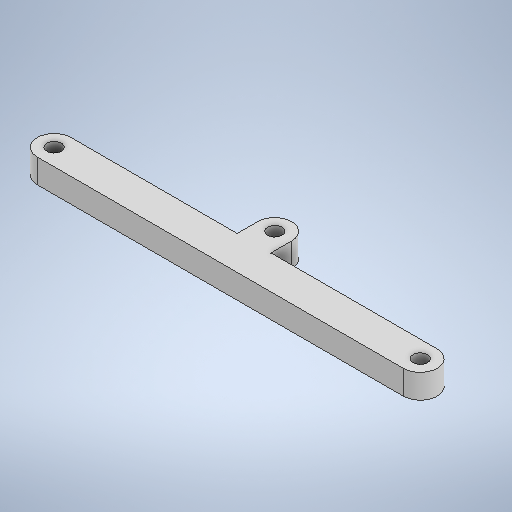
# Autodesk Inventor part: connector
Saved by Autodesk Inventor 2026 (Build 300175050, 175E)
## iProperties
Created: 2025-05-24
Part Number: connector
Material: Generic
Document SubType Name: Modeling
Designer: omiye
Density: 1 g/cm^3
Appearance: Default
Author: omiye
Autodesk Inventor part; units mm, degrees
ref_plane "YZ Plane" through (0, 0, 0) normal (1, 0, 0) x (0, 1, 0)
ref_plane "XZ Plane" through (0, 0, 0) normal (0, 1, 0) x (-1, 0, 0)
ref_plane "XY Plane" through (0, 0, 0) normal (0, 0, 1) x (1, 0, 0)
sketch "Sketch1" plane through (0, 0, 0) normal (0, 1, 0) x (-1, 0, 0)
  line L0 (-19, -3.5) -> (-19, 3.5)
  line L1 (-19, 3.5) -> (19, 3.5)
  line L2 (19, 3.5) -> (19, -3.5)
  line L3 (19, -3.5) -> (-19, -3.5)
  line L4 (-19, -3.5) -> (19, 3.5) construction
  line L5 (-19, 3.5) -> (19, -3.5) construction
  circle A0 centre (19, 0) radius 1.5
  line L6 (19, 3.5) -> (22.5, 3.5)
  line L7 (22.5, 3.5) -> (22.5, -3.5)
  line L8 (22.5, -3.5) -> (19, -3.5)
  line L9 (19, -3.5) -> (19, 3.5)
  line L10 (-19, 0) -> (-19, -7.8)
  line L11 (-22.5, 14.8) -> (-22.5, -7.8)
  line L12 (-22.5, -7.8) -> (-15.5, -7.8)
  line L13 (-15.5, -7.8) -> (-15.5, 14.8)
  line L14 (-15.5, 14.8) -> (-22.5, 14.8)
  line L15 (-22.5, 14.8) -> (-15.5, -7.8) construction
  line L16 (-22.5, -7.8) -> (-15.5, 14.8) construction
  line L17 (-19, 3.5) -> (-22.5, 3.5)
  circle A1 centre (-19, -7.8) radius 1.5
  line L18 (-15.5, -7.8) -> (-22.5, -7.8)
  line L19 (-22.5, -7.8) -> (-22.5, -11.3)
  line L20 (-22.5, -11.3) -> (-15.5, -11.3)
  line L21 (-15.5, -11.3) -> (-15.5, -7.8)
  point P0 (0, 0)
  point P1 (-22.5, -7.8)
  point P2 (-15.5, -3.5)
  dimension "d0" = 7
  dimension "d1" = 38
  dimension "d2" = 3
  dimension "d3" = 3.5
  dimension "d4" = 7.8
  dimension "d5" = 7
  dimension "d6" = 3
  dimension "d7" = 3.5
  constraints: 44 end point, 9 parallel, 7 midpoint, 4 perpendicular, 2 centre point, 2 horizontal, 1 coincident, 1 point on line, 1 vertical
  measures "d0" distance of L0.start L0.end
  measures "d1" distance of L0.end L1.end
  measures "d2" diameter of A0
  measures "d3" distance of L7.end L8.end
  measures "d4" distance of L10.start L10.end
  measures "d5" distance of L12.end L11.end
  measures "d6" diameter of A1
  measures "d7" distance of L19.end L18.end
extrude "Extrusion1" add sketch "Sketch1" along normal blind 5 contours L10 A1 L12 L11 L17 L0 | L0 L1 L13 L3 | L3 L13 L12 A1 L10 | L13 L1 L2 A0 L3 | L2 A0 L6 L7 L8 | L21 L20 L19 L12 A1
fillet "Fillet1" radius 3.5 5 edges at (22.5, 2.5, -11.3) (15.5, 2.5, -11.3) (22.5, 2.5, 3.5) (-22.5, 2.5, 3.5) (-22.5, 2.5, -3.5)
sketch "Sketch2" plane through (0, 5, 0) normal (0, 1, 0) x (1, 0, 0)
  arc A0 (19, -3.5) -> (22.5, 0) centre (19, 0) ccw projected
  line L0 (22.5, 0) -> (64, 0)
  line L1 (15.5, 3.5) -> (22.5, 3.5)
  line L2 (22.5, 3.5) -> (22.5, -3.5)
  line L3 (22.5, -3.5) -> (15.5, -3.5)
  line L4 (15.5, -3.5) -> (15.5, 3.5)
  line L5 (22.5, -3.5) -> (64, -3.5)
  line L6 (64, -3.5) -> (64, 3.5)
  line L7 (64, 3.5) -> (22.5, 3.5)
  line L8 (22.5, 3.5) -> (22.5, -3.5)
  line L9 (64, 3.5) -> (67.5, 3.5)
  line L10 (67.5, 3.5) -> (67.5, -3.5)
  line L11 (67.5, -3.5) -> (64, -3.5)
  line L12 (64, -3.5) -> (64, 3.5)
  circle A1 centre (64, 0) radius 1.65
  point P0 (0, 0)
  point P1 (22.5, 0)
  point P2 (19, -3.5)
  dimension "d11" = 41.5
  dimension "d12" = 3.5
  dimension "d13" = 3.3
  constraints: 26 end point, 6 parallel, 4 horizontal, 3 perpendicular, 2 point on line, 1 centre point, 1 coincident
  measures "d11" distance of L0.start L0.end
  measures "d12" distance of L10.end L11.end
  measures "d13" diameter of A1
extrude "Extrusion2" add sketch "Sketch2" against normal up to surface (5 mm away) contours A0 L2 L3 | L2 L7 L6 A1 L0 | L0 A1 L6 L5 L2 | L6 A1 L9 L10 L11
fillet "Fillet2" radius 3.5 2 edges at (67.5, 2.5, 3.5) (67.5, 2.5, -3.5)
sketch "Sketch3" plane through (0, 5, 0) normal (0, 1, 0) x (1, 0, 0)
  line L0 (19, 0) -> (57, 0)
  line L1 (19, 0) -> (60.5, 0)
  line L2 (19, 0) -> (60.5, 0) construction
  circle A0 centre (60.5, 0) radius 1.65
  point P0 (0, 0)
  dimension "d17" = 38
  dimension "d18" = 41.5
  dimension "d19" = 0
  dimension "d20" = 3.3
  constraints: 6 end point, 3 horizontal, 1 centre point, 1 coincident, 1 collinear
  measures "d17" distance of L0.start L0.end
  measures "d18" distance of L0.start L1.end
  measures "d19" distance between parallel lines of L1 L2
  measures "d20" diameter of A0
extrude "Extrusion3" cut sketch "Sketch3" against normal blind 10
sketch "Sketch4" plane through (0, 5, 0) normal (0, 1, 0) x (1, 0, 0)
  line L0 (-19, -3.5) -> (64, -3.5) projected
  line L1 (62.2745, -3.5) -> (67.2267, -3.5)
  line L2 (67.2267, -3.5) -> (67.2267, 3.993)
  line L3 (67.2267, 3.993) -> (62.2745, 3.993)
  line L4 (62.2745, 3.993) -> (62.2745, -3.5)
  line L5 (67.2267, 3.993) -> (67.8067, 3.993)
  line L6 (67.8067, 3.993) -> (67.8067, -3.5)
  line L7 (67.8067, -3.5) -> (67.2267, -3.5)
  line L8 (67.2267, -3.5) -> (67.2267, 3.993)
  point P0 (0, 0)
  constraints: 16 end point, 4 parallel, 2 horizontal, 2 perpendicular, 1 point on line
extrude "Extrusion4" cut sketch "Sketch4" against normal blind 10
sketch "Sketch5" plane through (0, 5, 0) normal (0, 1, 0) x (1, 0, 0)
  circle A0 centre (60.5, 0) radius 1.65 projected
  line L0 (60.5, 0) -> (64, 0)
  line L1 (-19, -3.5) -> (62.2745, -3.5) projected
  line L2 (60.5, -3.5) -> (64, -3.5)
  line L3 (64, -3.5) -> (64, 3.5)
  line L4 (64, 3.5) -> (60.5, 3.5)
  line L5 (60.5, 3.5) -> (60.5, -3.5)
  point P0 (0, 0)
  point P1 (60.5, 1.65)
  point P2 (60.5, -1.65)
  dimension "d25" = 3.5
  dimension "d26" = 7
  constraints: 10 end point, 2 horizontal, 2 parallel, 1 perpendicular, 1 point on line
  measures "d25" distance of L0.start L0.end
  measures "d26" distance of L3.end L2.end
extrude "Extrusion5" add sketch "Sketch5" against normal up to surface (5 mm away) contours L0 L3 L2 L1 L5 A0 | A0 L5 L4 L3 L0
fillet "Fillet3" radius 3.5 2 edges at (64, 2.5, 3.5) (64, 2.5, -3.5)
sketch "Sketch6" plane through (0, 5, 0) normal (0, 1, 0) x (1, 0, 0)
  circle A0 centre (19, 7.8) radius 1.5 projected
  line L0 (19, 7.8) -> (19, 0)
  circle A1 centre (-19, 0) radius 1.5 projected
  line L1 (19, 0) -> (-19, 0)
  line L2 (-19, 0) -> (19, 0)
  line L3 (19, 0) -> (57, 0)
  line L4 (60.5, 3.5) -> (22.5, 3.5) projected
  line L5 (57, 3.5) -> (64.573, 3.5)
  line L6 (64.573, 3.5) -> (64.573, -3.5)
  line L7 (64.573, -3.5) -> (57, -3.5)
  line L8 (57, -3.5) -> (57, 3.5)
  point P0 (0, 0)
  dimension "d30" = 38
  constraints: 16 end point, 3 equal length, 2 perpendicular, 2 point on line, 1 horizontal, 1 vertical
  measures "d30" distance of L0.end L3.end
extrude "Extrusion6" add sketch "Sketch6" against normal up to surface (5 mm away) contours L5 L6 L7 L8 L4
sketch "Sketch7" plane through (0, 5, 0) normal (0, 1, 0) x (1, 0, 0)
  circle A0 centre (19, 7.8) radius 1.5 projected
  line L0 (19, 7.8) -> (19, 0)
  line L1 (19, 0) -> (57, 0)
  circle A1 centre (57, 0) radius 1.5
  line L2 (57, 0) -> (60.5, 0)
  line L3 (-19, -3.5) -> (64.573, -3.5) projected
  line L4 (64.573, 3.5) -> (22.5, 3.5) projected
  line L5 (60.5, -3.5) -> (64.573, -3.5)
  line L6 (64.573, -3.5) -> (64.573, 3.5)
  line L7 (64.573, 3.5) -> (60.5, 3.5)
  line L8 (60.5, 3.5) -> (60.5, -3.5)
  point P0 (0, 0)
  point P1 (64.573, -3.5)
  dimension "d33" = 7.8
  dimension "d34" = 38
  dimension "d35" = 3
  dimension "d36" = 3.5
  constraints: 14 end point, 2 horizontal, 2 parallel, 2 perpendicular, 1 centre point, 1 coincident, 1 point on line, 1 vertical
  measures "d33" distance of L0.start L0.end
  measures "d34" distance of L0.end L1.end
  measures "d35" diameter of A1
  measures "d36" distance of L2.start L2.end
extrude "Extrusion7" cut sketch "Sketch7" against normal blind 10 contours A1 L2 L1 | L1 L2 A1 | L8 L4 L6 L3
fillet "Fillet4" radius 3.5 2 edges at (60.5, 2.5, -3.5) (60.5, 2.5, 3.5)
body "Solid1"
